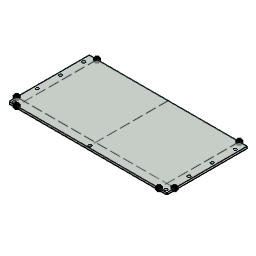
Rear Panel - BLANK (Autodesk Fusion 360 design; units mm, degrees)
Autodesk Fusion 360 part; units mm, degrees
sketch "Sketch1" plane through (0, 0, 0) normal (0, 0, 1) x (1, 0, 0)
  line L0 (-121.3, 61.7) -> (121.3, 61.7)
  line L1 (121.3, 61.7) -> (121.3, -61.7)
  line L2 (121.3, -61.7) -> (-121.3, -61.7)
  line L3 (-121.3, -61.7) -> (-121.3, 61.7)
  point P0 (0, 61.7)
  point P1 (-121.3, 0)
  dimension "d1" = 123.4
  dimension "d2" = 242.6
  constraint horizontal L0
  constraint vertical L1
  constraint horizontal L2
  constraint vertical L3
  constraint midpoint L0 P0
  constraint midpoint L3 P1
  constraint vertical origin P0
  constraint horizontal origin P1
  measures "d1" distance of L0.end L1.end
  measures "d2" distance of L0.start L0.end
extrude "Extrude1" add sketch "Sketch1" along normal blind 3
sketch "Sketch2" plane through (0, 0, 3) normal (0, 0, 1) x (-1, 0, 0)
  line L0 (121.3, 61.7) -> (-121.3, 61.7)
  line L1 (-121.3, 61.7) -> (-121.3, -61.7)
  line L2 (-121.3, -61.7) -> (121.3, -61.7)
  line L3 (121.3, -61.7) -> (121.3, 61.7)
  line L4 (0, -61.7) -> (0, 61.7) construction
  circle A0 centre (116.5, -48.5) radius 2.25
  circle A1 centre (116.5, -12.9) radius 2.25
  circle A2 centre (116.5, 22.7) radius 2.25
  circle A3 centre (116.5, 58.3) radius 2.25
  circle A4 centre (0, 58.3) radius 2.25
  circle A5 centre (-116.5, -48.5) radius 2.25
  circle A6 centre (-116.5, -12.9) radius 2.25
  circle A7 centre (-116.5, 22.7) radius 2.25
  circle A8 centre (-116.5, 58.3) radius 2.25
  dimension "d5" = 4.5
  dimension "d6" = 4.5
  dimension "d7" = 4.5
  dimension "d8" = 4.5
  dimension "d9" = 4.5
  dimension "d10" = 4.5
  dimension "d11" = 4.5
  dimension "d12" = 4.5
  dimension "d13" = 4.5
  dimension "d15" = 233
  dimension "d16" = 13.2
  dimension "d17" = 35.6
  dimension "d18" = 35.6
  dimension "d71" = 35.6
  constraint midpoint L2 L4.start
  constraint midpoint L0 L4.end
  constraint vertical A0.centre A1.centre
  constraint vertical A1.centre A2.centre
  constraint vertical A2.centre A3.centre
  constraint vertical A5.centre A6.centre
  constraint vertical A6.centre A7.centre
  constraint vertical A7.centre A8.centre
  constraint horizontal A0.centre A5.centre
  constraint horizontal A1.centre A6.centre
  constraint horizontal A2.centre A7.centre
  constraint horizontal A3.centre A4.centre
  constraint horizontal A4.centre A8.centre
  constraint symmetric L4 A0.centre A5.centre
  constraint coincident L4 A4.centre
  measures "d5" diameter of A0
  measures "d6" diameter of A1
  measures "d7" diameter of A2
  measures "d8" diameter of A3
  measures "d9" diameter of A5
  measures "d10" diameter of A6
  measures "d11" diameter of A7
  measures "d12" diameter of A8
  measures "d13" diameter of A4
  measures "d15" distance of A0.centre A5.centre
  measures "d16" distance of L2 A0.centre
  measures "d17" distance of A0.centre A1.centre
  measures "d18" distance of A1.centre A2.centre
  measures "d71" distance of A2.centre A3.centre
extrude "Extrude2" cut sketch "Sketch2" against normal blind 3 contours A0 | A1 | A2 | A3 | A4 | A5 | A6 | A7 | A8
fillet "Fillet1" radius 1 2 edges at (121.3, -61.7, 1.5) (-121.3, -61.7, 1.5)
sketch "Sketch3" plane through (0, 0, 0) normal (0, 0, -1) x (1, 0, 0)
  circle A0 centre (116.5, 22.7) radius 2.25
  circle A1 centre (-116.5, 22.7) radius 2.25
  circle A2 centre (-116.5, -12.9) radius 2.25
  circle A3 centre (116.5, 58.3) radius 2.25
  circle A4 centre (116.5, -12.9) radius 2.25
  circle A5 centre (-116.5, 58.3) radius 2.25
  circle A6 centre (-116.5, -48.5) radius 2.25
  circle A7 centre (0, 58.3) radius 2.25
  circle A8 centre (116.5, -48.5) radius 2.25
  arc A9 (-120.3, 61.7) -> (-121.3, 60.7) centre (-120.3, 60.7) ccw
  line L0 (-121.3, 60.7) -> (-121.3, -61.7)
  line L1 (-121.3, -61.7) -> (121.3, -61.7)
  line L2 (121.3, -61.7) -> (121.3, 60.7)
  arc A10 (121.3, 60.7) -> (120.3, 61.7) centre (120.3, 60.7) ccw
  line L3 (120.3, 61.7) -> (-120.3, 61.7)
  line L4 (121.3, -58.5) -> (118.9588, -58.5)
  line L5 (118.9588, -58.5) -> (-121.3, -58.5) construction
  line L6 (111.1, -61.7) -> (111.1, 61.7)
  line L7 (-111.1, -61.7) -> (-111.1, 61.7)
  line L8 (0, -61.7) -> (0, 61.7) construction
  line L9 (111.1, -58.5) -> (-111.1, -58.5)
  line L10 (-111.1, -58.5) -> (-111.1, -54.5)
  line L11 (-111.1, -54.5) -> (111.1, -54.5)
  line L12 (111.1, -54.5) -> (111.1, -58.5)
  dimension "d23" = 3.2
  dimension "d24" = 10.2
  dimension "d25" = 3.2
  dimension "d26" = 4
  constraint coincident L2 L4.start
  constraint perpendicular L2 L4
  constraint coincident L0 L5.end
  constraint perpendicular L0 L5
  constraint coincident L1 L6.start
  constraint coincident L3 L6.end
  constraint perpendicular L3 L6
  constraint coincident L1 L7.start
  constraint coincident L3 L7.end
  constraint perpendicular L3 L7
  constraint midpoint L1 L8.start
  constraint midpoint L3 L8.end
  constraint symmetric L6 L7 L8
  constraint horizontal L9
  constraint vertical L10
  constraint horizontal L11
  constraint vertical L12
  constraint coincident L7 L10.end
  constraint coincident L6 L9.start
  measures "d23" distance of L1 L5
  measures "d24" distance of L2 L6
  measures "d25" distance of L1 L9
  measures "d26" distance of L5 L11
extrude "Extrude3" add sketch "Sketch3" along normal blind 8 contours L6 L7 L9 L10 L11 L12
chamfer "Chamfer1" distance 8 angle 45 1 edges at (0, 54.5, 0)
sketch "Sketch4" plane through (0, 58.5, 0) normal (0, 1, 0) x (-1, 0, 0)
  line L0 (111.1, 0) -> (-111.1, 0)
  line L1 (-111.1, 0) -> (-111.1, -8)
  line L2 (-111.1, -8) -> (111.1, -8)
  line L3 (111.1, -8) -> (111.1, 0)
  line L4 (-111.1, -4) -> (111.1, -4) construction
  circle A0 centre (-40.165, -4) radius 1.95
  circle A1 centre (40.165, -4) radius 1.95
  line L5 (0, 0) -> (0, -8) construction
  dimension "d30" = 3.9
  dimension "d31" = 3.9
  dimension "d34" = 80.33
  dimension "d35" = 70.935
  dimension "d36" = 70.935
  constraint midpoint L1 L4.start
  constraint midpoint L3 L4.end
  constraint coincident L4 A0.centre
  constraint coincident L4 A1.centre
  constraint coincident L5.start origin
  constraint midpoint L2 L5.end
  constraint symmetric A0 A1 L5
  measures "d30" diameter of A0
  measures "d31" diameter of A1
  measures "d34" distance of A0.centre A1.centre
  measures "d35" distance of L3 A1.centre
  measures "d36" distance of L1 A0.centre
extrude "Extrude4" cut sketch "Sketch4" against normal blind 12 contours A0 | A1
fillet "Fillet2" radius 2 2 edges at (-111.1, 56.5, -8) (111.1, 56.5, -8)
sketch "Sketch1 (1)" plane through (0, 0, 3) normal (0, 0, 1) x (-1, 0, 0)
  arc A0 (121.3, 60.7) -> (120.3, 61.7) centre (120.3, 60.7) ccw
  line L0 (120.3, 61.7) -> (-120.3, 61.7)
  arc A1 (-120.3, 61.7) -> (-121.3, 60.7) centre (-120.3, 60.7) ccw
  line L1 (-121.3, 60.7) -> (-121.3, -61.7)
  line L2 (-121.3, -61.7) -> (121.3, -61.7)
  line L3 (121.3, -61.7) -> (121.3, 60.7)
  circle A2 centre (-116.5, 22.7) radius 2.25
  circle A3 centre (116.5, 22.7) radius 2.25
  circle A4 centre (116.5, -12.9) radius 2.25
  circle A5 centre (-116.5, 58.3) radius 2.25
  circle A6 centre (-116.5, -12.9) radius 2.25
  circle A7 centre (116.5, 58.3) radius 2.25
  circle A8 centre (116.5, -48.5) radius 2.25
  circle A9 centre (0, 58.3) radius 2.25
  circle A10 centre (-116.5, -48.5) radius 2.25
  line L4 (-121.3, 49.7) -> (-116.2313, 49.7)
  line L5 (-116.2313, 49.7) -> (121.3, 49.7) construction
  line L6 (-109.3, -61.7) -> (-109.3, 61.7) construction
  line L7 (109.3, -61.7) -> (109.3, 61.7) construction
  line L8 (0, -61.7) -> (0, 61.7) construction
  dimension "d38" = 12
  dimension "d39" = 12
  constraint coincident L1 L4.start
  constraint perpendicular L1 L4
  constraint coincident L3 L5.end
  constraint perpendicular L3 L5
  constraint coincident L2 L6.start
  constraint coincident L0 L6.end
  constraint perpendicular L0 L6
  constraint coincident L2 L7.start
  constraint coincident L0 L7.end
  constraint perpendicular L0 L7
  constraint midpoint L2 L8.start
  constraint midpoint L0 L8.end
  constraint symmetric L6 L7 L8
  measures "d38" distance of L0 L5
  measures "d39" distance of L3 L7
equation "d6 = d5"
equation "d7 = d5"
equation "d8 = d5"
equation "d9 = d5"
equation "d10 = d5"
equation "d11 = d5"
equation "d12 = d5"
equation "d13 = d5"
equation "d31 = d30"
equation "d71 = d18"
